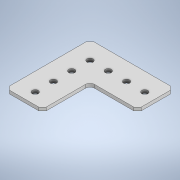
# Autodesk Inventor part: ShortenedVersaGusset 90o
Saved by Autodesk Inventor 2022 (Build 260153000, 153)
## iProperties
Created: 2020-01-14
Part Number: ShortenedVersaGusset 90o
Material: Generic
Document SubType Name: Modeling
Designer: aidan
Density: 1 g/cm^3
Appearance: Default
Author: aidan
Autodesk Inventor part; units mm, degrees
ref_plane "YZ Plane" through (0, 0, 0) normal (1, 0, 0) x (0, 1, 0)
ref_plane "XZ Plane" through (0, 0, 0) normal (0, 1, 0) x (-1, 0, 0)
ref_plane "XY Plane" through (0, 0, 0) normal (0, 0, 1) x (1, 0, 0)
sketch "Sketch1" plane through (0, 0, 0) normal (0, 1, 0) x (-1, 0, 0)
  line L0 (38.4325, -41.9578) -> (13.0325, -41.9578)
  line L1 (13.0325, -41.9578) -> (13.0325, 16.4622)
  line L2 (13.0325, 16.4622) -> (38.4325, 16.4622)
  line L3 (38.4325, 16.4622) -> (38.4325, -41.9578)
  line L4 (38.4325, -41.9578) -> (-9.6784, 6.153) construction
  line L5 (38.4325, -41.9578) -> (38.4325, -16.5578)
  line L6 (38.4325, -16.5578) -> (-19.9875, -16.5578)
  line L7 (-19.9875, -16.5578) -> (-19.9875, -41.9578)
  line L8 (-19.9875, -41.9578) -> (38.4325, -41.9578)
  point P0 (0, 0)
  point P1 (13.0325, -16.5578)
  dimension "d0" = 25.4
  dimension "d1" = 58.42
  dimension "d2" = 45
  constraints: 18 end point, 3 symmetric about line, 2 parallel, 1 horizontal, 1 perpendicular
  measures "d0" distance of L0.start L0.end
  measures "d1" distance of L2.end L0.start
  measures "d2" angle of L0 L4
extrude "Extrusion1" add sketch "Sketch1" along normal blind 2.286
chamfer "Chamfer1" distance 2.54 angle 45 1 edges at (-13.0325, 1.143, 16.4622)
chamfer "Chamfer2" distance 2.54 angle 45 4 edges at (-38.4325, 1.143, 16.4622) (19.9875, 1.143, -16.5578) (19.9875, 1.143, -41.9578) (-38.4325, 1.143, -41.9578)
fillet "Fillet1" radius 3.175 1 edges at (-13.0325, 1.143, -16.5578)
sketch "Sketch2" plane through (0, 2.286, 0) normal (0, 1, 0) x (1, 0, 0)
  circle A0 centre (-25.8595, 29.3848) radius 2.0828
  line L0 (17.4475, 41.9578) -> (-35.8925, 41.9578) projected
  line L1 (19.9875, 19.0978) -> (19.9875, 39.4178) projected
  line L2 (-38.4325, 39.4178) -> (-38.4325, -13.9222) projected
  point P0 (0, 0)
  dimension "d12" = 12.573
  dimension "d14" = 4.1656
  dimension "d23" = 12.573
  constraints: 1 centre point
  measures "d12" distance from line of L0 A0.centre
  measures "d14" diameter of A0
  measures "d23" distance from line of A0.centre L2
extrude "Extrusion2" cut sketch "Sketch2" against normal blind 2.286
pattern_linear "Rectangular Pattern1" count 5 spacing 12.7 along (0, 0, 1) of "Extrusion2"
pattern_linear "Rectangular Pattern2" count 5 spacing 12.7 along (1, 0, 0) of "Extrusion2"
body "Solid1"
